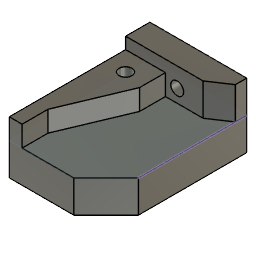
Design 1 Robocon Task 3 (Autodesk Fusion 360 design; units mm, degrees)
part number: 2026-03-05-20-25-14-190
Autodesk Fusion 360 part; units mm, degrees
note: some values were not read from the file. Set by a fixed rule: which sketch regions a step uses.
sketch "Sketch1" plane through (0, 0, 0) normal (0, 0, 1) x (1, 0, 0)
  line L0 (-50, 0) -> (0, 0)
  line L1 (25, 25) -> (0, 0)
  line L2 (-50, 0) -> (-50, 140)
  line L3 (21.9831, 108.8475) -> (-62.7657, 108.8475)
  line L4 (-50, 108.8475) -> (-62.7657, 108.8475)
  line L5 (25, 25) -> (25, 110)
  line L6 (21.9831, 108.8475) -> (25, 108.8475)
  constraint coincident L0.end L1.end
  constraint horizontal L0
  constraint perpendicular L0 L2
  constraint perpendicular L2 L3
  constraint coincident L2 L4.start
  constraint coincident L3 L4.start
  constraint vertical L5
  constraint coincident L5 L6.end
  constraint perpendicular L5 L6
extrude "Extrude1" add sketch "Sketch1" along normal blind 25
sketch "Sketch2" plane through (0, 0, 25) normal (0, 0, 1) x (-1, 0, 0)
  line L0 (-25, -108.8475) -> (50, -108.8475)
  line L1 (50, -108.8475) -> (50, 0)
  line L2 (50, 0) -> (0, 0)
  line L3 (0, 0) -> (-25, -25)
  line L4 (-25, -25) -> (-25, -108.8475)
sketch "Sketch3" plane through (0, 0, 25) normal (0, 0, 1) x (-1, 0, 0)
  line L0 (-10, -90) -> (-25, -97)
  line L1 (-25, -108.8475) -> (-25, -97)
  line L2 (-10, -90) -> (50, -90)
  line L3 (19.1012, -90) -> (19.1012, -70)
  line L4 (19.1012, -70) -> (40, -20)
  line L5 (40, -20) -> (40, 0)
  line L6 (40, 0) -> (50, 0)
  line L7 (50, 0) -> (50, -108.8475)
  line L8 (50, -90) -> (50, -108.8475)
  line L9 (-25, -97) -> (-25, -108.8475)
  line L10 (50, -108.8475) -> (50, -90)
  point P0 (-25, -108.8475)
  point P1 (50, 0)
  point P2 (50, -108.8475)
  constraint coincident P0 L1.start
  constraint coincident L2 L3.start
  constraint perpendicular L2 L3
  constraint parallel L3 L5
  constraint coincident P1 L6.end
  constraint perpendicular L5 L6
  constraint coincident P2 L7.end
  constraint coincident L2.end L8.start
extrude "Extrude2" add sketch "Sketch3" along normal blind 16
sketch "Sketch4" plane through (0, 0, 25) normal (0, 0, 1) x (-1, 0, 0)
  line L0 (-10, -90) -> (-25, -100)
  line L1 (-25, -108.8475) -> (-25, -100)
  line L2 (-25, -108.8475) -> (50, -108.8475)
  line L3 (50, -108.8475) -> (50, -90)
  line L4 (50, -90) -> (-10, -90)
  point P0 (-25, -108.8475)
  point P1 (50, -108.8475)
  constraint coincident P0 L1.start
  constraint coincident P1 L2.end
  constraint perpendicular L2 L3
  constraint perpendicular L3 L4
extrude "Extrude3" add sketch "Sketch4" along normal blind 25
sketch "Sketch5" plane through (0, 0, 41) normal (0, 0, 1) x (-1, 0, 0)
  line L0 (19.1012, -90) -> (50, -90)
  line L1 (50, -90) -> (50, 0)
  line L2 (50, 0) -> (40, 0)
  line L3 (40, 0) -> (40, -20)
  line L4 (40, -20) -> (19.1012, -70)
  line L5 (19.1012, -70) -> (19.1012, -90)
  circle A0 centre (35, -75) radius 5
extrude "Extrude4" cut sketch "Sketch5" against normal blind 41 contours A0
sketch "Sketch6" plane through (0, 90, 0) normal (0, -1, 0) x (1, 0, 0)
  line L0 (-50, 41) -> (-19.1012, 41)
  line L1 (-19.1012, 41) -> (-19.1012, 25)
  line L2 (-19.1012, 25) -> (10, 25)
  line L3 (10, 25) -> (10, 50)
  line L4 (10, 50) -> (-50, 50)
  line L5 (-50, 50) -> (-50, 41)
  circle A0 centre (-10, 35) radius 5
  dimension "d11" = 10
  measures "d11" diameter of A0
extrude "Extrude5" cut sketch "Sketch6" against normal blind 25 contours A0
